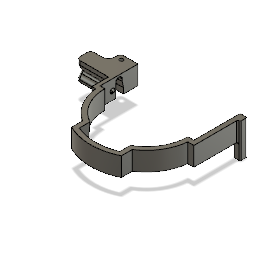
Base_Led (Autodesk Fusion 360 design; units mm, degrees)
Autodesk Fusion 360 part; units mm, degrees
sketch "Sketch1" plane through (0, 0, 0) normal (0, 1, 0) x (1, 0, 0)
  line L0 (-40, 7) -> (-40, -0.0001)
  line L1 (-40, -0.0001) -> (-35, -0.0001)
  arc A0 (-35, -0.0001) -> (-17, -30.5941) centre (0, 0) ccw
  line L2 (-17, -30.5941) -> (-17, -39.4968)
  arc A1 (-17, -39.4968) -> (0, -43) centre (0, 0) ccw
  line L3 (0, -1.75) -> (0, -22.5)
  arc A2 (0, -43) -> (17, -39.4968) centre (0, 0) ccw
  line L4 (17, -30.5941) -> (17, -39.4968)
  arc A3 (17, -30.5941) -> (35, -0.0001) centre (0, 0) ccw
  line L5 (40, -0.0001) -> (35, -0.0001)
  line L6 (40, 7) -> (40, -0.0001)
  line L7 (40, 7) -> (-40, 7)
  arc A4 (0, -47) -> (21, -42.0476) centre (0, 0) ccw
  line L8 (21, -32.8634) -> (21, -42.0476)
  arc A5 (21, -32.8634) -> (38.7943, -4.0001) centre (0, 0) ccw
  line L9 (44, -4.0001) -> (38.7943, -4.0001)
  line L10 (44, 11) -> (44, -4.0001)
  line L11 (44, 11) -> (-44, 11)
  line L12 (-44, 11) -> (-44, -4.0001)
  line L13 (-44, -4.0001) -> (-38.7943, -4.0001)
  arc A6 (-38.7943, -4.0001) -> (-21, -32.8634) centre (0, 0) ccw
  line L14 (-21, -32.8634) -> (-21, -42.0476)
  arc A7 (-21, -42.0476) -> (0, -47) centre (0, 0) ccw
  line L15 (-40, 7) -> (-44, 7)
  line L16 (40, 7) -> (44, 7)
  line L17 (-39, 7) -> (-39, -0.0001)
  line L18 (-39, 7) -> (-39, 31.9999)
  line L19 (-44, 11) -> (-44, 31.9999)
  line L20 (-39, 31.9999) -> (-44, 31.9999)
  line L21 (-44, -4.0001) -> (-69, -4.0001)
  line L22 (-69, -4.0001) -> (-69, 31.9999)
  line L23 (-69, 31.9999) -> (-44, 31.9999)
  line L24 (-44, 31.9999) -> (-44, -4.0001)
  line L25 (0, 0) -> (50, 0)
  dimension "d1" = 40
  dimension "d2" = 35
  dimension "d3" = 17
  dimension "d4" = 43
  dimension "d5" = 4
  dimension "d8" = 1
  dimension "d11" = 32
  dimension "d12" = 30
  dimension "d90" = 7
  constraint vertical L0
  constraint perpendicular L0 L1
  constraint coincident A0.centre A1.centre
  constraint vertical L2
  constraint symmetric A0.centre L3 A1.centre
  constraint symmetric L0.start L3 L6.start
  constraint symmetric L0.end L3 L5.start
  constraint symmetric L1.end L3 A3.end
  constraint symmetric A0.end L3 L4.start
  constraint symmetric A0 L3 A3
  constraint symmetric L2.end L3 A2.end
  constraint symmetric A1.end L3 A2.start
  constraint symmetric A1 L3 A2
  constraint coincident L12 L15.end
  constraint perpendicular L12 L15
  constraint coincident L10 L16.end
  constraint perpendicular L10 L16
  constraint coincident L7 L17.start
  constraint coincident L1 L17.end
  constraint perpendicular L1 L17
  constraint perpendicular L7 L18
  constraint perpendicular L11 L19
  constraint perpendicular L19 L20
  constraint horizontal L21
  constraint vertical L22
  constraint horizontal L23
  constraint vertical L24
  constraint horizontal L25
  constraint collinear L20 L23
  measures "d1" distance of A0.centre L0
  measures "d2" radius of A0
  measures "d3" distance of L2 A0.centre
  measures "d4" radius of A1
  measures "d8" distance of L0 L17
  measures "d11" distance of L1 L20
  measures "d12" distance of L18 L22
  measures "d90" distance of L16 L25
extrude "Extrude1" add sketch "Sketch1" along normal blind 16 contours L0 L1 L7 L17 | L7 L11 L12 L15 L18 L24 | L0 L1 A0 L2 A1 A2 L4 A3 L5 A4 L8 A5 L9 L10 L12 L13 A6 L14 A7 L15 L24 L25 | L12 L19 L21 L22 L23 L24 | L6 L10 L16 L25 | L11 L18 L19 L20 L24
draft "Draft1" angle -7.5 neutral plane through (0, 16, 0) pull (0, 1, 0) 2 faces at (-17, 10.6667, 33.5617) (17, 5.3333, 33.5617)
ref_plane "WorkPlane1" through (-37, 8, -15.9999) normal (0, 0, -1) x (-1, 0, 0)
sketch "Sketch2" plane through (-54, 8, -15.9999) normal (0, 0, -1) x (1, 0, 0)
  line L0 (15, -6.5) -> (7, -6.5)
  line L1 (7, -6.5) -> (7, -3.75)
  line L2 (7, -3.75) -> (15, -3.75)
  line L3 (15, -3.75) -> (15, -6.5)
  line L4 (15, 8) -> (15, -8)
  line L5 (7, -3.75) -> (6, -3.75)
  line L6 (6, -3.75) -> (6, -6.75)
  line L7 (6, -6.75) -> (7, -6.75)
  line L8 (7, -6.75) -> (7, -3.75)
  line L9 (15, -8) -> (-15, -8)
  line L10 (-4.3794, -3.75) -> (-4, -3.75) construction
  line L11 (-4, -3.75) -> (29.236, -3.75) construction
  dimension "d14" = 1.5
  dimension "d15" = 2.75
  dimension "d16" = 3
  dimension "d17" = 8
  dimension "d18" = 1
  constraint horizontal L0
  constraint vertical L1
  constraint horizontal L2
  constraint vertical L3
  constraint coincident L0.start L4
  constraint horizontal L5
  constraint vertical L6
  constraint horizontal L7
  constraint vertical L8
  constraint perpendicular L6 L10
  constraint perpendicular L6 L11
  constraint collinear L2 L11
  measures "d14" distance of L0 L9
  measures "d15" distance of L0.start L2.end
  measures "d16" distance of L5.end L6.end
  measures "d17" distance of L0.start L0.end
  measures "d18" distance of L6.end L7.end
revolve "Revolve1" cut sketch "Sketch2" angle 90 about axis through (-58, 11.75, -15.9999) along (-1, 0, 0) second angle 90
extrude "Extrude2" cut 1 faces at (-44.3333, 11.75, -15.0832) along direction (0, -1, 0) through all
sketch "Sketch3" plane through (0, 0, 0) normal (0, -1, 0) x (1, 0, 0)
  line L0 (-39, -18.7499) -> (-47, -18.7499)
  line L1 (-47, -18.7499) -> (-47, -18.9999)
  line L2 (-47, -18.9999) -> (-48, -18.9999)
  line L3 (-48, -18.9999) -> (-48, -12.9999)
  line L4 (-48, -12.9999) -> (-47, -12.9999)
  line L5 (-47, -12.9999) -> (-47, -13.2499)
  line L6 (-47, -13.2499) -> (-39, -13.2499)
  line L7 (-39, -13.2499) -> (-39, 0.0001)
  line L8 (-39, 0.0001) -> (-35, 0.0001)
  arc A0 (-19.1064, 29.3248) -> (-35, 0.0001) centre (0, 0) ccw
  line L9 (-19.1064, 29.3248) -> (-19.1064, 38.522)
  arc A1 (19.1064, 38.522) -> (-19.1064, 38.522) centre (0, 0) ccw
  line L10 (19.1064, 38.522) -> (19.1064, 29.3248)
  arc A2 (35, 0.0001) -> (19.1064, 29.3248) centre (0, 0) ccw
  line L11 (35, 0.0001) -> (40, 0.0001)
  line L12 (40, 0.0001) -> (40, -7)
  line L13 (40, -7) -> (44, -7)
  line L14 (44, -7) -> (44, 4.0001)
  line L15 (44, 4.0001) -> (38.7943, 4.0001)
  arc A3 (38.7943, 4.0001) -> (21, 32.8634) centre (0, 0) ccw
  line L16 (21, 32.8634) -> (21, 42.0476)
  arc A4 (21, 42.0476) -> (-21, 42.0476) centre (0, 0) ccw
  line L17 (-21, 42.0476) -> (-21, 32.8634)
  arc A5 (-21, 32.8634) -> (-38.7943, 4.0001) centre (0, 0) ccw
  line L18 (-38.7943, 4.0001) -> (-69, 4.0001)
  line L19 (-69, 4.0001) -> (-69, -31.9999)
  line L20 (-69, -31.9999) -> (-39, -31.9999)
  line L21 (-39, -31.9999) -> (-39, -18.7499)
  line L22 (-49.1462, -11.9999) -> (-66, -11.9999)
  line L23 (-66, -11.9999) -> (-66, -19.9999)
  line L24 (-66, -19.9999) -> (-49.1462, -19.9999)
  line L25 (-49.1462, -19.9999) -> (-49.1462, -11.9999)
  line L26 (-39, -13.2499) -> (-39, -18.7499) construction
  line L27 (-39, -15.9999) -> (-93, -15.9999) construction
  line L28 (-39, -18.7499) -> (-50, -18.7499) construction
  line L29 (-39, -13.2499) -> (-50, -13.2499) construction
  line L30 (-48, -13.2499) -> (-49.1462, -13.2499)
  line L31 (-48, -18.7499) -> (-49.1462, -18.7499)
  line L32 (-48, -18.7499) -> (-48, -13.2499)
  dimension "d23" = 3
  dimension "d24" = 8
  constraint horizontal L22
  constraint vertical L23
  constraint horizontal L24
  constraint vertical L25
  constraint midpoint L26 L27.start
  constraint perpendicular L19 L27
  constraint midpoint L23 L27
  constraint coincident L0.start L21.end
  constraint perpendicular L25 L28
  constraint coincident L6.end L7.start
  constraint perpendicular L7 L29
  constraint coincident L3 L30.start
  constraint coincident L29 L30.start
  constraint coincident L25 L30.end
  constraint coincident L29 L30.end
  constraint coincident L3 L31.start
  constraint coincident L28 L31.start
  constraint coincident L28 L31.end
  constraint coincident L25 L31.end
  measures "d23" distance of L19 L23
  measures "d24" distance of L22.end L23.end
extrude "Extrude3" cut sketch "Sketch3" against normal blind 13 contours L3 L25 L30 L31 L32 | L22 L23 L24 L25
sketch "Sketch4" plane through (0, 0, 0) normal (0, -1, 0) x (1, 0, 0)
  line L0 (-48, -18.7499) -> (-49.1462, -18.7499)
  line L1 (-49.1462, -18.7499) -> (-49.1462, -19.9999)
  line L2 (-49.1462, -19.9999) -> (-66, -19.9999)
  line L3 (-66, -19.9999) -> (-66, -11.9999)
  line L4 (-66, -11.9999) -> (-49.1462, -11.9999)
  line L5 (-49.1462, -11.9999) -> (-49.1462, -13.2499)
  line L6 (-49.1462, -13.2499) -> (-48, -13.2499)
  line L7 (-48, -13.2499) -> (-48, -12.9999)
  line L8 (-48, -12.9999) -> (-47, -12.9999)
  line L9 (-47, -12.9999) -> (-47, -13.2499)
  line L10 (-47, -13.2499) -> (-39, -13.2499)
  line L11 (-39, -13.2499) -> (-39, 0.0001)
  line L12 (-39, 0.0001) -> (-35, 0.0001)
  arc A0 (-19.1064, 29.3248) -> (-35, 0.0001) centre (0, 0) ccw
  line L13 (-19.1064, 29.3248) -> (-19.1064, 38.522)
  arc A1 (19.1064, 38.522) -> (-19.1064, 38.522) centre (0, 0) ccw
  line L14 (19.1064, 38.522) -> (19.1064, 29.3248)
  arc A2 (35, 0.0001) -> (19.1064, 29.3248) centre (0, 0) ccw
  line L15 (35, 0.0001) -> (40, 0.0001)
  line L16 (40, 0.0001) -> (40, -7)
  line L17 (40, -7) -> (44, -7)
  line L18 (44, -7) -> (44, 4.0001)
  line L19 (44, 4.0001) -> (38.7943, 4.0001)
  arc A3 (38.7943, 4.0001) -> (21, 32.8634) centre (0, 0) ccw
  line L20 (21, 32.8634) -> (21, 42.0476)
  arc A4 (21, 42.0476) -> (-21, 42.0476) centre (0, 0) ccw
  line L21 (-21, 42.0476) -> (-21, 32.8634)
  arc A5 (-21, 32.8634) -> (-38.7943, 4.0001) centre (0, 0) ccw
  line L22 (-38.7943, 4.0001) -> (-69, 4.0001)
  line L23 (-69, 4.0001) -> (-69, -31.9999)
  line L24 (-69, -31.9999) -> (-39, -31.9999)
  line L25 (-39, -31.9999) -> (-39, -18.7499)
  line L26 (-39, -18.7499) -> (-47, -18.7499)
  line L27 (-47, -18.7499) -> (-47, -18.9999)
  line L28 (-47, -18.9999) -> (-48, -18.9999)
  line L29 (-48, -18.9999) -> (-48, -18.7499)
  line L30 (-69, 4.0001) -> (-42, 4.0001)
  line L31 (-42, 4.0001) -> (-42, -9.9999)
  line L32 (-42, -9.9999) -> (-69, -9.9999)
  line L33 (-69, -9.9999) -> (-69, 4.0001)
  dimension "d27" = 3
  dimension "d28" = 2
  constraint horizontal L30
  constraint vertical L31
  constraint horizontal L32
  constraint vertical L33
  constraint coincident L22.end L23.start
  measures "d27" distance of L11 L31
  measures "d28" distance of L4 L32
extrude "Extrude4" cut sketch "Sketch4" against normal blind 19 contours L22 L23 L30 L31 L32 L33
sketch "Sketch5" plane through (-39, 0, 0) normal (1, 0, 0) x (0, 0, -1)
  line L0 (31.9999, 16) -> (-0.0001, 16)
  arc A0 (18.7499, 11.75) -> (13.2499, 11.75) centre (15.9999, 11.75) ccw
  circle A1 centre (10.4999, 7) radius 2
  line L1 (18.7499, 11.75) -> (18.7499, 0)
  line L2 (18.7499, 0) -> (31.9999, 0)
  line L3 (31.9999, 0) -> (31.9999, 16)
  line L4 (-0.0001, 16) -> (-0.0001, 0)
  line L5 (-0.0001, 0) -> (13.2499, 0)
  line L6 (13.2499, 0) -> (13.2499, 11.75)
  dimension "d34" = 9
  dimension "d35" = 4
  dimension "d83" = 10.5
  measures "d34" distance of L0 A1.centre
  measures "d35" diameter of A1
  measures "d83" distance of A1.centre L4
extrude "Extrude5" cut sketch "Sketch5" against normal blind 44 contours A1
extrude "Extrude6" add 1 faces at (-49.1462, 1.8924, -12.4166) along direction (-1, 0, 0) blind 17
fillet "Fillet1" radius 4.5 1 edges at (-55.5, 5.0635, -9.9999)
ref_plane "WorkPlane2" through (-12.5, 5, 10.2679) normal (0, -1, 0) x (-1, 0, 0)
sketch "Sketch11" plane through (-39, 0, 0) normal (1, 0, 0) x (0, 0, -1)
  line L0 (18.7499, 11.75) -> (18.7499, 0)
  line L1 (18.7499, 0) -> (31.9999, 0)
  line L2 (31.9999, 0) -> (31.9999, 16)
  line L3 (31.9999, 16) -> (-0.0001, 16)
  line L4 (-0.0001, 16) -> (-0.0001, 0)
  line L5 (-0.0001, 0) -> (13.2499, 0)
  line L6 (13.2499, 0) -> (13.2499, 11.75)
  arc A0 (18.7499, 11.75) -> (13.2499, 11.75) centre (15.9999, 11.75) ccw
  line L7 (18.7499, 0) -> (19.7499, 0)
  line L8 (19.7499, 0) -> (19.7499, 9.75)
  line L9 (19.7499, 9.75) -> (18.7499, 9.75)
  line L10 (18.7499, 9.75) -> (18.7499, 0)
  circle A1 centre (10.4999, 7) radius 2
  dimension "d64" = 2
  dimension "d65" = 1
  constraint horizontal L7
  constraint vertical L8
  constraint horizontal L9
  constraint vertical L10
  constraint coincident L0.end L1.start
  measures "d64" distance of L0.start L9.end
  measures "d65" distance of L8.end L9.end
extrude "Extrude12" cut sketch "Sketch11" against normal blind 11 contours L0 L1 L7 L8 L9 L10
chamfer "Chamfer2" distance 5 distance2 1 1 edges at (-44.0731, 9.75, -19.7499) measured on face at (-42.3821, 3.25, -19.7499)
extrude "Extrude13" add 1 faces at (41.3333, 5.3333, -7) along direction (0, 0, -1) blind 30
sketch "Sketch12" plane through (0, 0, 0) normal (0, -1, 0) x (1, 0, 0)
  line L0 (-39, -19.7499) -> (-49.1462, -19.7499)
  line L1 (-49.1462, -19.7499) -> (-49.1462, -19.9999)
  line L2 (-49.1462, -19.9999) -> (-66, -19.9999)
  line L3 (-66, -19.9999) -> (-66, -13.2499)
  line L4 (-66, -13.2499) -> (-48, -13.2499)
  line L5 (-48, -13.2499) -> (-48, -12.9999)
  line L6 (-48, -12.9999) -> (-47, -12.9999)
  line L7 (-47, -12.9999) -> (-47, -13.2499)
  line L8 (-47, -13.2499) -> (-39, -13.2499)
  line L9 (-39, -13.2499) -> (-39, 0.0001)
  line L10 (-39, 0.0001) -> (-35, 0.0001)
  arc A0 (-19.1064, 29.3248) -> (-35, 0.0001) centre (0, 0) ccw
  line L11 (-19.1064, 29.3248) -> (-19.1064, 38.522)
  arc A1 (19.1064, 38.522) -> (-19.1064, 38.522) centre (0, 0) ccw
  line L12 (19.1064, 38.522) -> (19.1064, 29.3248)
  arc A2 (35, 0.0001) -> (19.1064, 29.3248) centre (0, 0) ccw
  line L13 (35, 0.0001) -> (40, 0.0001)
  line L14 (40, 0.0001) -> (40, -37)
  line L15 (40, -37) -> (44, -37)
  line L16 (44, -37) -> (44, 4.0001)
  line L17 (44, 4.0001) -> (38.7943, 4.0001)
  arc A3 (38.7943, 4.0001) -> (21, 32.8634) centre (0, 0) ccw
  line L18 (21, 32.8634) -> (21, 42.0476)
  arc A4 (21, 42.0476) -> (-21, 42.0476) centre (0, 0) ccw
  line L19 (-21, 42.0476) -> (-21, 32.8634)
  arc A5 (-21, 32.8634) -> (-38.7943, 4.0001) centre (0, 0) ccw
  line L20 (-38.7943, 4.0001) -> (-42, 4.0001)
  line L21 (-42, 4.0001) -> (-42, -9.9999)
  line L22 (-42, -9.9999) -> (-69, -9.9999)
  line L23 (-69, -9.9999) -> (-69, -31.9999)
  line L24 (-69, -31.9999) -> (-39, -31.9999)
  line L25 (-39, -31.9999) -> (-39, -19.7499)
  line L26 (-69, -31.9999) -> (-54, -31.9999)
  line L27 (-54, -31.9999) -> (-54, -21.9999)
  line L28 (-54, -21.9999) -> (-69, -21.9999)
  line L29 (-69, -21.9999) -> (-69, -31.9999)
  dimension "d72" = 2
  dimension "d73" = 15
  constraint horizontal L26
  constraint vertical L27
  constraint horizontal L28
  constraint vertical L29
  constraint coincident L23.end L24.start
  measures "d72" distance of L2 L28
  measures "d73" distance of L23.end L26.end
extrude "Extrude14" cut sketch "Sketch12" against normal blind 16 contours L23 L24 L26 L27 L28 L29
fillet "Fillet5" radius 5 1 edges at (-54, 8, -21.9999)
sketch "Sketch13" plane through (0, 0, 0) normal (0, -1, 0) x (1, 0, 0)
  line L0 (-54, -31.9999) -> (-39, -31.9999)
  line L1 (-39, -31.9999) -> (-39, -19.7499)
  line L2 (-39, -19.7499) -> (-49.1462, -19.7499)
  line L3 (-49.1462, -19.7499) -> (-49.1462, -19.9999)
  line L4 (-49.1462, -19.9999) -> (-66, -19.9999)
  line L5 (-66, -19.9999) -> (-66, -13.2499)
  line L6 (-66, -13.2499) -> (-48, -13.2499)
  line L7 (-48, -13.2499) -> (-48, -12.9999)
  line L8 (-48, -12.9999) -> (-47, -12.9999)
  line L9 (-47, -12.9999) -> (-47, -13.2499)
  line L10 (-47, -13.2499) -> (-39, -13.2499)
  line L11 (-39, -13.2499) -> (-39, 0.0001)
  line L12 (-39, 0.0001) -> (-35, 0.0001)
  arc A0 (-19.1064, 29.3248) -> (-35, 0.0001) centre (0, 0) ccw
  line L13 (-19.1064, 29.3248) -> (-19.1064, 38.522)
  arc A1 (19.1064, 38.522) -> (-19.1064, 38.522) centre (0, 0) ccw
  line L14 (19.1064, 38.522) -> (19.1064, 29.3248)
  arc A2 (35, 0.0001) -> (19.1064, 29.3248) centre (0, 0) ccw
  line L15 (35, 0.0001) -> (40, 0.0001)
  line L16 (44, 4.0001) -> (38.7943, 4.0001)
  arc A3 (38.7943, 4.0001) -> (21, 32.8634) centre (0, 0) ccw
  line L17 (21, 32.8634) -> (21, 42.0476)
  arc A4 (21, 42.0476) -> (-21, 42.0476) centre (0, 0) ccw
  line L18 (-21, 42.0476) -> (-21, 32.8634)
  arc A5 (-21, 32.8634) -> (-38.7943, 4.0001) centre (0, 0) ccw
  line L19 (-38.7943, 4.0001) -> (-42, 4.0001)
  line L20 (-42, 4.0001) -> (-42, -9.9999)
  line L21 (-42, -9.9999) -> (-69, -9.9999)
  line L22 (-69, -9.9999) -> (-69, -21.9999)
  line L23 (-69, -21.9999) -> (-59, -21.9999)
  arc A6 (-54, -26.9999) -> (-59, -21.9999) centre (-59, -26.9999) ccw
  line L24 (-54, -26.9999) -> (-54, -31.9999)
  line L25 (40, -33) -> (46, -33)
  line L26 (46, -33) -> (46, -39)
  line L27 (46, -39) -> (40, -39)
  line L28 (40, -39) -> (40, -33)
  line L29 (40, 0.0001) -> (40, -37)
  line L30 (44, -37) -> (40, -37)
  dimension "d108" = 6
  dimension "d109" = 2
  dimension "d110" = 6
  constraint horizontal L25
  constraint vertical L26
  constraint horizontal L27
  constraint vertical L28
  constraint coincident L25.start L29
  measures "d108" distance of L25.end L26.end
  measures "d109" distance of L27 L30
  measures "d110" distance of L25.start L25.end
fillet "Fillet7" radius 5.5 1 edges at (-55.5, 8.9365, -9.9999)
fillet "Fillet8" radius 2.5 1 edges at (-42, 7.0668, -8.501)
fillet "Fillet9" radius 3 7 edges at (-69, 8, -21.9999) (-54, 8, -31.9999) (-69, 14.2951, -9.9999) (-69, 10.3448, -10.4791) (-69, 6.9332, -12.4988) (-69, 3.8499, -10.4557) (-69, 0.9383, -9.9999)
extrude "Extrude16" add sketch "Sketch13" along normal blind 14 and the other way blind 16
fillet "Fillet10" radius 1 2 edges at (42, 0, -33) (44, 8, -33)
chamfer "Chamfer5" distance 1 angle 45 4 edges at (46, -14, -36) (43, -14, -33) (40, -14, -36) (43, -14, -39)
fillet "Fillet11" radius 1 6 edges at (40, 1.5, -39) (46, 1.5, -39) (46, 1.5, -33) (40, -7, -33) (40, -0.2929, -32.7071) (40, 0, -15.9999)
sketch "Sketch15" plane through (0, 0, 0) normal (0, -1, 0) x (1, 0, 0)
  line L0 (41, 0.0001) -> (41, -32)
  line L1 (41, -32) -> (44, -32)
  line L2 (44, -32) -> (44, 4.0001)
  line L3 (44, 4.0001) -> (38.7943, 4.0001)
  arc A0 (38.7943, 4.0001) -> (21, 32.8634) centre (0, 0) ccw
  line L4 (21, 32.8634) -> (21, 42.0476)
  arc A1 (21, 42.0476) -> (-21, 42.0476) centre (0, 0) ccw
  line L5 (-21, 42.0476) -> (-21, 32.8634)
  arc A2 (-21, 32.8634) -> (-38.7943, 4.0001) centre (0, 0) ccw
  line L6 (-38.7943, 4.0001) -> (-42, 4.0001)
  line L7 (-42, 4.0001) -> (-42, -9.9999)
  line L8 (-42, -9.9999) -> (-66, -9.9999)
  arc A3 (-66, -9.9999) -> (-69, -12.9999) centre (-66, -12.9999) ccw
  line L9 (-69, -12.9999) -> (-69, -18.9999)
  arc A4 (-69, -18.9999) -> (-66, -21.9999) centre (-66, -18.9999) ccw
  line L10 (-66, -21.9999) -> (-59, -21.9999)
  arc A5 (-54, -26.9999) -> (-59, -21.9999) centre (-59, -26.9999) ccw
  line L11 (-54, -26.9999) -> (-54, -28.9999)
  arc A6 (-54, -28.9999) -> (-51, -31.9999) centre (-51, -28.9999) ccw
  line L12 (-51, -31.9999) -> (-39, -31.9999)
  line L13 (-39, -31.9999) -> (-39, -19.7499)
  line L14 (-39, -19.7499) -> (-49.1462, -19.7499)
  line L15 (-49.1462, -19.7499) -> (-49.1462, -19.9999)
  line L16 (-49.1462, -19.9999) -> (-66, -19.9999)
  line L17 (-66, -19.9999) -> (-66, -13.2499)
  line L18 (-66, -13.2499) -> (-48, -13.2499)
  line L19 (-48, -13.2499) -> (-48, -12.9999)
  line L20 (-48, -12.9999) -> (-47, -12.9999)
  line L21 (-47, -12.9999) -> (-47, -13.2499)
  line L22 (-47, -13.2499) -> (-39, -13.2499)
  line L23 (-39, -13.2499) -> (-39, 0.0001)
  line L24 (-39, 0.0001) -> (-35, 0.0001)
  arc A7 (-19.1064, 29.3248) -> (-35, 0.0001) centre (0, 0) ccw
  line L25 (-19.1064, 29.3248) -> (-19.1064, 38.522)
  arc A8 (19.1064, 38.522) -> (-19.1064, 38.522) centre (0, 0) ccw
  line L26 (19.1064, 38.522) -> (19.1064, 29.3248)
  arc A9 (35, 0.0001) -> (19.1064, 29.3248) centre (0, 0) ccw
  line L27 (35, 0.0001) -> (41, 0.0001)
  circle A10 centre (-49, -28) radius 1.55
  dimension "d114" = 28
  dimension "d115" = 49
  dimension "d116" = 3.1
  measures "d114" vertical distance of A0.centre A10.centre
  measures "d115" horizontal distance of A0.centre A10.centre
  measures "d116" diameter of A10
extrude "Extrude18" cut sketch "Sketch15" against normal blind 16 contours A10
